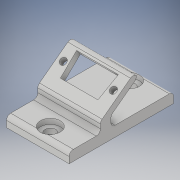
# Autodesk Inventor part: D-SUB-9POL
Saved by Autodesk Inventor 2019 (Build 230136000, 136)
## iProperties
Created: 2018-05-12
Part Number: D-SUB-9POL
Material: Generisch
Document SubType Name: Modeling
Designer: marc
Density: 1 g/cm^3
Appearance: Vorgabe
Author: marc
## iProperties of the stored document D-SUB-9POL_3D-Druck.ipt
Created: 2018-05-12
Part Number: D-SUB-9POL_3D-Druck
Material: Generisch
Document SubType Name: Modeling
Designer: marc
Density: 1 g/cm^3
Appearance: Vorgabe
Author: marc
Autodesk Inventor part; units mm, degrees
ref_plane "YZ Plane" through (0, 0, 0) normal (1, 0, 0) x (0, 1, 0)
ref_plane "XZ Plane" through (0, 0, 0) normal (0, 1, 0) x (-1, 0, 0)
ref_plane "XY Plane" through (0, 0, 0) normal (0, 0, 1) x (1, 0, 0)
sketch "Skizze1" plane through (0, 0, 0) normal (0, 1, 0) x (-1, 0, 0)
  line L0 (0, 0) -> (30, 0)
  line L1 (30, 0) -> (30, 50)
  line L2 (30, 50) -> (0, 50)
  line L3 (0, 50) -> (0, 0)
  dimension "d0" = 30
  dimension "d1" = 50
  constraints: 8 end point, 2 parallel, 1 horizontal, 1 perpendicular
  measures "d0" distance of L2.end L1.end
  measures "d1" distance of L1.end L0.end
extrude "Extrusion1" add sketch "Skizze1" along normal blind 5
sketch "Skizze2" plane through (0, 5, 0) normal (0, 1, 0) x (1, 0, 0)
  line L0 (-30, -50) -> (0, -50) projected
  line L1 (-30, 0) -> (-30, -50) projected
  line L2 (0, 0) -> (-30, 0) projected
  point P0 (-15, -44)
  point P1 (-15, -6)
  dimension "d4" = 6
  dimension "d5" = 15
  dimension "d6" = 15
  dimension "d7" = 6
  measures "d4" distance from line of L0 point (-15, -44)
  measures "d5" distance from line of L1 point (-15, -44)
  measures "d6" distance from line of L1 point (-15, -6)
  measures "d7" distance from line of L2 point (-15, -6)
hole "Bohrung1" at (-15, 5, 44) at (-15, 5, 6) direction (0, -1, 0) diameter 5.1 end through all counterbore diameter 9.5 counterbore depth 2.5
sketch "Skizze3" plane through (0, 5, 0) normal (0, 1, 0) x (1, 0, 0)
  line L0 (-30, -35) -> (0, -35)
  line L1 (0, -35) -> (0, -30)
  line L2 (0, -30) -> (-30, -30)
  line L3 (-30, -30) -> (-30, -35)
  line L4 (-30, 0) -> (-30, -50) projected
  line L5 (-30, -50) -> (0, -50) projected
  point P0 (0, 0)
  dimension "d15" = 30
  dimension "d16" = 5
  dimension "d17" = 15
  constraints: 8 end point, 2 parallel, 1 horizontal, 1 perpendicular, 1 point on line
  measures "d15" distance of L2.end L1.end
  measures "d16" distance between parallel lines of L2 L0
  measures "d17" distance between parallel lines of L5 L0
extrude "Extrusion2" add sketch "Skizze3" along normal blind 5
sketch "Skizze4" plane through (0, 0, 50) normal (1, 0, 0) x (0, 0, -1)
  line L0 (15, 5) -> (15, 10) projected
  line L1 (15, 10) -> (31, 22)
  line L2 (31, 22) -> (32.8, 19.6)
  line L3 (20, 5) -> (20, 10) projected
  line L4 (32.8, 19.6) -> (20, 10)
  line L5 (20, 10) -> (15, 10)
  point P0 (50, 0)
  dimension "d20" = 20
  dimension "d21" = 3
  constraints: 8 end point, 3 perpendicular
  measures "d20" distance of L0.end L1.end
  measures "d21" distance of L1.end L2.end
extrude "Extrusion3" add sketch "Skizze4" against normal up to surface (30 mm away)
sketch "Skizze5" plane through (-30, 10, 35) normal (0, 0.8, 0.6) x (1, 0, 0)
  line L0 (6, 6) -> (24, 6)
  line L1 (24, 6) -> (25, 17)
  line L2 (25, 17) -> (5, 17)
  line L3 (6, 6) -> (5, 17)
  line L4 (30, 20) -> (0, 20) projected
  line L5 (0, 0) -> (0, 20) projected
  line L6 (30, 0) -> (30, 20) projected
  point P0 (30, 22)
  dimension "d24" = 18
  dimension "d25" = 20
  dimension "d26" = 1
  dimension "d27" = 3
  dimension "d28" = 11
  dimension "d29" = 5
  dimension "d30" = 5
  constraints: 8 end point, 1 horizontal, 1 parallel
  measures "d24" distance of L0.start L0.end
  measures "d25" distance of L1.end L2.end
  measures "d26" horizontal distance of L1.end L0.end
  measures "d27" distance between parallel lines of L4 L2
  measures "d28" distance between parallel lines of L2 L0
  measures "d29" distance from line of L5 L2.end
  measures "d30" distance from line of L6 L1.end
extrude "Extrusion4" cut sketch "Skizze5" against normal up to surface (3 mm away)
sketch "Skizze6" plane through (-30, 10, 35) normal (0, 0.8, 0.6) x (1, 0, 0)
  line L0 (5, 17) -> (25, 17) projected
  line L1 (24, 6) -> (6, 6) projected
  line L2 (30, 0) -> (30, 20) projected
  line L3 (0, 0) -> (0, 20) projected
  point P0 (30, 22)
  point P1 (3, 11.5)
  point P2 (27, 11.5)
  dimension "d33" = 11
  dimension "d34" = 5.5
  dimension "d35" = 3
  dimension "d36" = 5.5
  dimension "d37" = 3
  measures "d33" distance between parallel lines of L0 L1
  measures "d34" distance from line of L0 point (27, 11.5)
  measures "d35" distance from line of L2 point (27, 11.5)
  measures "d36" vertical distance of L0.start point (3, 11.5)
  measures "d37" distance from line of L3 point (3, 11.5)
hole "Bohrung2" at (-27, 16.9, 25.8) at (-3, 16.9, 25.8) direction (0, -0.8, -0.6) diameter 3.1 depth 8 tip angle 118
fillet "Rundung1" radius 2 8 edges at (-15, 10, 35) (-15, 5, 50) (-15, 5, 0) (-15, 22, 19) (-15, 19.6, 17.2) (-15, 10, 30) (-15, 5, 30) (-15, 5, 35)
equation "\"d6\" = d5"
equation "\"d7\" = d4"
equation "\"d34\" = 0.5 * d33"
equation "\"d36\" = d34"
equation "\"d37\" = d35"
